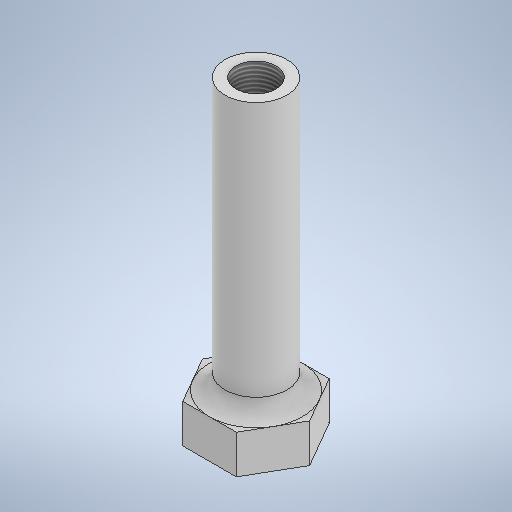
# Autodesk Inventor part: zamkniecie_sworzenia_2
Saved by Autodesk Inventor 2025.2 (Build 292293000, 293)
## iProperties
Created: 2025-11-27
Part Number: zamkniecie_sworzenia_2
Material: Ogólny
Document SubType Name: Modeling
Designer: juras
Density: 1 g/cm^3
Appearance: Domyślna
Author: juras
Autodesk Inventor part; units mm, degrees
ref_plane "YZ Plane" through (0, 0, 0) normal (1, 0, 0) x (0, 1, 0)
ref_plane "XZ Plane" through (0, 0, 0) normal (0, 1, 0) x (-1, 0, 0)
ref_plane "XY Plane" through (0, 0, 0) normal (0, 0, 1) x (1, 0, 0)
sketch "Szkic1" plane through (0, 0, 0) normal (0, 1, 0) x (-1, 0, 0)
  circle A0 centre (0, 0) radius 4
  dimension "d0" = 8
  constraints: 1 centre point, 1 coincident
  measures "d0" diameter of A0
extrude "Wyciągnięcie proste1" add sketch "Szkic1" along normal mid plane 35
sketch "Szkic2" plane through (0, 17.5, 0) normal (0, 1, 0) x (1, 0, 0)
  circle A0 centre (0, 0) radius 2.6
  dimension "d3" = 5.2
  constraints: 1 centre point, 1 coincident
  measures "d3" diameter of A0
extrude "Wyciągnięcie proste2" cut sketch "Szkic2" against normal blind 25
thread "Gwint1" size "M5.5x0.5" class "6H" standard "ANSI Metric M Profile" length 25
sketch "Szkic3" plane through (0, -17.5, 0) normal (0, -1, 0) x (1, 0, 0)
  line L0 (3.4641, 6) -> (6.9282, 0)
  line L1 (6.9282, 0) -> (3.4641, -6)
  line L2 (3.4641, -6) -> (-3.4641, -6)
  line L3 (-3.4641, -6) -> (-6.9282, 0)
  line L4 (-6.9282, 0) -> (-3.4641, 6)
  line L5 (-3.4641, 6) -> (3.4641, 6)
  point P0 (0, 0)
  point P1 (0, 0)
  dimension "d8" = 6
  dimension "d10" = 6
  constraints: 12 end point, 1 coincident, 13 other
  measures "d8" distance from line of point (0, 0) L5
  measures "d10" vertical distance of L0.end L1.end
extrude "Wyciągnięcie proste3" add sketch "Szkic3" along normal blind 5
fillet "Zaokrąglenie1" radius 2 1 edges at (4, -17.5, 0)
